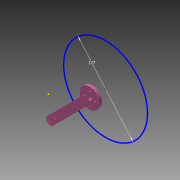
# Autodesk Inventor part: Arm2
Saved by Autodesk Inventor 2015 (Build 190159000, 159)
## iProperties
Created: 2017-01-13
Part Number: Arm2
Material: Generic
Document SubType Name: Modeling
Designer: Per
Density: 1 g/cm^3
Appearance: Pink
Author: Per
Autodesk Inventor part; units mm, degrees
ref_plane "YZ Plane" through (0, 0, 0) normal (1, 0, 0) x (0, 1, 0)
ref_plane "XZ Plane" through (0, 0, 0) normal (0, 1, 0) x (-1, 0, 0)
ref_plane "XY Plane" through (0, 0, 0) normal (0, 0, 1) x (1, 0, 0)
sketch "Sketch1" plane through (0, 0, 0) normal (0, 1, 0) x (-1, 0, 0)
  arc A0 (-71.9329, 45.7909) -> (-81.9156, 35.8082) centre (-86.283, 50.1583) ccw
  circle A1 centre (-25.4718, -10.6529) radius 1.5
  line L0 (-24.7647, -15.6026) -> (-20.5221, -11.36)
  line L1 (-24.7647, -15.6026) -> (-29.0074, -15.6026)
  line L2 (-20.5221, -11.36) -> (-20.5221, -7.1174)
  circle A2 centre (-33.25, -2.8747) radius 1.5
  circle A3 centre (-86.283, 40.6583) radius 1.5
  circle A4 centre (-94.283, 50.1583) radius 1.5
  circle A5 centre (-86.283, 59.6583) radius 1.5
  circle A6 centre (-78.283, 50.1583) radius 1.5
  circle A7 centre (-86.283, 50.1583) radius 3
  line L3 (-71.4338, 43.7943) -> (-20.5221, -7.1174)
  line L4 (-29.0074, -15.6026) -> (-79.919, 35.309)
  arc A8 (-71.9329, 45.7909) -> (-71.4338, 43.7943) centre (-70.0196, 45.2085) ccw
  arc A9 (-79.919, 35.309) -> (-81.9156, 35.8082) centre (-81.3333, 33.8948) ccw
  point P0 (0, 0)
  point P1 (-18.4008, -9.2387)
  point P2 (-72.3193, 44.6798)
  point P3 (-80.8045, 36.1945)
  point P4 (-26.886, -17.724)
  point P5 (-72.3193, 44.6798)
  dimension "d2" = 3
  dimension "d3" = 3
  dimension "d4" = 3
  dimension "d6" = 6
  dimension "d10" = 2
  constraints: 10 centre point, 10 end point, 8 point on circle, 4 point on line, 4 tangent, 1 coincident, 1 equal radius, 1 parallel
  measures "d2" diameter of A3
  measures "d3" diameter of A4
  measures "d4" diameter of A5
  measures "d6" diameter of A7
  measures "d10" radius of A8
extrude "Arm 4 mm" add sketch "Sketch1" along normal blind 4
ref_plane "Simulerar Motor" through (0, 24, 0) normal (0, 1, 0) x (1, 0, 0)
sketch "Propeller" plane through (0, 24, 0) normal (0, 1, 0) x (1, 0, 0)
  circle A0 centre (86.283, -50.1583) radius 63.5
  point P0 (0, 0)
  dimension "d14" = 127
  constraints: 1 centre point, 1 coincident
  measures "d14" diameter of A0
body "Solid2"
